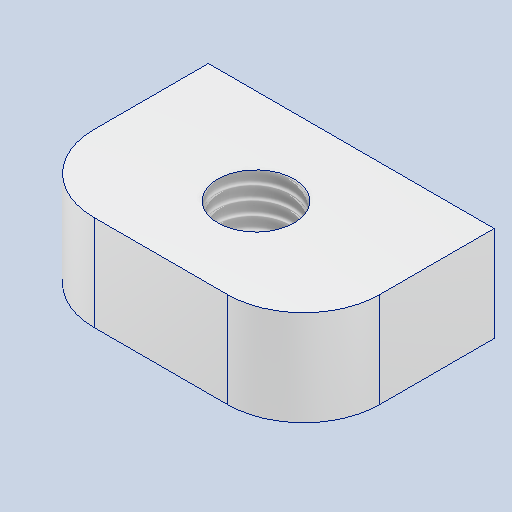
# Autodesk Inventor part: víko_držák
Saved by Autodesk Inventor 2023 (Build 270158000, 158)
## iProperties
Created: 2023-04-03
Part Number: víko_držák
Material: Aluminum 6061
Document SubType Name: Modeling
Designer: lukyv
Density: 2.7 g/cm^3
Appearance: Aluminum - Flat
Mass: 1.76265 g
Surface Area: 5.56796 cm^2
Volume: 0.652832 cm^3
Author: lukyv
Autodesk Inventor part; units mm, degrees
ref_plane "YZ Plane" through (0, 0, 0) normal (1, 0, 0) x (0, 1, 0)
ref_plane "XZ Plane" through (0, 0, 0) normal (0, 1, 0) x (-1, 0, 0)
ref_plane "XY Plane" through (0, 0, 0) normal (0, 0, 1) x (1, 0, 0)
sketch "Sketch1" plane through (0, 0, 0) normal (0, 0, 1) x (1, 0, 0)
  line L0 (30.1319, -27.3816) -> (15.1319, -27.3816)
  line L1 (15.1319, -27.3816) -> (15.1319, -32.3816)
  line L2 (15.1319, -32.3816) -> (30.1319, -32.3816)
  line L3 (30.1319, -32.3816) -> (30.1319, -27.3816)
  point P0 (0, 0)
  dimension "d0" = 15
  dimension "d1" = 5
  constraints: 8 end point, 2 parallel, 1 horizontal, 1 perpendicular
  measures "d0" distance of L2.end L1.end
  measures "d1" distance of L1.end L0.end
extrude "Extrusion1" add sketch "Sketch1" along normal blind 10
fillet "Fillet1" radius 4 2 edges at (15.1319, -29.8816, 10) (30.1319, -29.8816, 10)
sketch "Sketch2" plane through (15.1319, -27.3816, 0) normal (0, 1, 0) x (1, 0, 0)
  circle A0 centre (7.5, -5) radius 2
  line L0 (11, -10) -> (4, -10) projected
  line L1 (0, 0) -> (0, -6) projected
  point P0 (-15.1319, 0)
  dimension "d5" = 4
  dimension "d6" = 5
  dimension "d7" = 7.5
  constraints: 1 centre point
  measures "d5" diameter of A0
  measures "d6" distance from line of A0.centre L0
  measures "d7" distance from line of A0.centre L1
extrude "Extrusion2" cut sketch "Sketch2" against normal blind 7.5
thread "Thread1" size "M4x0.7" class "6H" standard "ANSI Metric M Profile" full length
body "Solid1"
